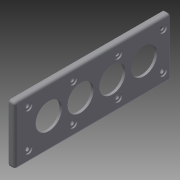
# Autodesk Inventor part: 160409 Sensor cover A_Miniature - A_Miniature - A_Miniature - A_Miniature - R23
Saved by Autodesk Inventor 2015 (Build 190159000, 159)
## iProperties
Created: 2016-02-28
Part Number: 160409 Sensor cover A_Miniature - A_Miniature - A_Miniature - A_Miniature - R23
Material: Generic
Document SubType Name: Modeling
Designer: gerbomi
Density: 1 g/cm^3
Appearance: Default
Author: gerbomi
Autodesk Inventor part; units mm, degrees
sketch "Sketch1" plane through (0, 0, 0) normal (0, 1, 0) x (-1, 0, 0)
  line L0 (2, 0) -> (102, 0)
  line L1 (104, -2) -> (104, -123)
  line L2 (102, -125) -> (2, -125)
  line L3 (0, -123) -> (0, -2)
  arc A0 (104, -2) -> (102, 0) centre (102, -2) ccw
  arc A1 (102, -125) -> (104, -123) centre (102, -123) ccw
  arc A2 (0, -123) -> (2, -125) centre (2, -123) ccw
  arc A3 (2, 0) -> (0, -2) centre (2, -2) ccw
  point P0 (0, 0)
  point P1 (104, -125)
  point P2 (0, -125)
  dimension "d0" = 104
  dimension "d1" = 125
  dimension "d2" = 2
  dimension "d3" = 2
  constraints: 8 end point, 8 point on circle, 8 tangent, 6 point on line, 4 centre point, 2 equal radius, 2 parallel, 1 horizontal, 1 perpendicular
  measures "d0" distance of point (104, -125) point (0, -125)
  measures "d1" distance of point (0, -125) point (0, 0)
  measures "d2" radius of A0
  measures "d3" radius of A3
extrude "Boîte extérieure" [suppressed]
fillet "Fillet1-Boîte extérieure" [suppressed]
ref_plane "Work Plane2 - PCB Vertical" through (0, 0, -62.5) normal (0, 0, 1) x (1, 0, 0)
ref_plane "Work Plane4 - Surface extérieure capteurs" through (0, 20.1, 0) normal (0, 1, 0) x (-1, 0, 0)
ref_plane "Work Plane6 - Fond creusé" through (0, 17, 0) normal (0, 1, 0) x (-1, 0, 0)
sketch "Sketch26" plane through (0, 20.1, 0) normal (0, 1, 0) x (-1, 0, 0)
  line L0 (16, -121) -> (36, -121)
  line L1 (47, -110) -> (47, -13)
  line L2 (36, -2) -> (16, -2)
  line L3 (5, -13) -> (5, -110)
  arc A0 (5, -110) -> (16, -121) centre (16, -110) ccw
  arc A1 (36, -121) -> (47, -110) centre (36, -110) ccw
  arc A2 (47, -13) -> (36, -2) centre (36, -13) ccw
  arc A3 (16, -2) -> (5, -13) centre (16, -13) ccw
  line L4 (0, -2) -> (0, -123) projected
  line L5 (0, -2) -> (0, -123) projected
  line L6 (104, -123) -> (104, -2) projected
  line L7 (2, -125) -> (102, -125) projected
  point P0 (0, 0)
  point P1 (47, -2)
  point P2 (47, -121)
  point P3 (5, -2)
  dimension "d158" = 42
  dimension "d159" = 119
  dimension "d160" = 11
  dimension "d161" = 5
  dimension "d186" = 4
  constraints: 8 end point, 8 point on circle, 8 tangent, 6 point on line, 4 centre point, 3 equal radius, 2 parallel, 1 horizontal, 1 perpendicular
  measures "d158" distance of point (5, -2) point (47, -2)
  measures "d159" distance of point (47, -2) point (47, -121)
  measures "d160" radius of A0
  measures "d161" distance between parallel lines of L4 L3
  measures "d186" distance between parallel lines of L7 L0
extrude "Centreur Echantillonnage actif" [suppressed]
sketch "Sketch 22" plane through (0, 17, 0) normal (0, 1, 0) x (-1, 0, 0)
  circle A0 centre (25.1, -19.83) radius 16.5
  line L0 (99, -5) -> (99, -120) projected
  line L1 (9, -5) -> (99, -5) projected
  circle A1 centre (25.1, -47.135) radius 10.5
  circle A2 centre (25.1, -72.535) radius 10.5
  circle A3 centre (25.1, -99.84) radius 16.5
  line L2 (102, 0) -> (2, 0) projected
  line L3 (0, -2) -> (0, -123) projected
  line L4 (2, -125) -> (102, -125) projected
  point P0 (0, 0)
  point P1 (99, -12.0721)
  point P2 (99, -58.79)
  point P3 (16.07, -5)
  point P4 (91.93, -5)
  dimension "d124" = 33
  dimension "d126" = 14.83
  dimension "d140" = 21
  dimension "d141" = 27.305
  dimension "d142" = 21
  dimension "d143" = 25.4
  dimension "d144" = 33
  dimension "d145" = 27.305
  dimension "d196" = 73.9
  dimension "d258" = 19.83
  dimension "d259" = 25.1
  dimension "d260" = 25.16
  constraints: 4 centre point
  measures "d124" diameter of A0
  measures "d126" distance from line of L1 A0.centre
  measures "d140" diameter of A1
  measures "d141" distance of A0.centre A1.centre
  measures "d142" diameter of A2
  measures "d143" distance of A1.centre A2.centre
  measures "d144" diameter of A3
  measures "d145" distance of A2.centre A3.centre
  measures "d196" distance from line of L0 A0.centre
  measures "d258" distance from line of L2 A0.centre
  measures "d259" distance from line of A0.centre L3
  measures "d260" distance from line of L4 A3.centre
extrude "Sensor A/Miniature or Sensoric" [suppressed]
sketch "Sketch35" plane through (0, 20.1, 0) normal (0, 1, 0) x (-1, 0, 0)
  circle A0 centre (40.5, -114) radius 1
  line L0 (47, -110) -> (47, -13) projected
  line L1 (16, -121) -> (36, -121) projected
  point P0 (0, 0)
  dimension "d235" = 2
  dimension "d244" = 6.5
  dimension "d245" = 7
  constraints: 1 centre point
  measures "d235" diameter of A0
  measures "d244" distance from line of L0 A0.centre
  measures "d245" distance from line of L1 A0.centre
extrude "Vis Centreur Chapeau" [suppressed]
pattern_linear "Rectangular Pattern3" [suppressed]
ref_plane "Work Plane10 - Chapeau ext." through (0, 25.1, 0) normal (0, 1, 0) x (-1, 0, 0)
sketch "Sketch36" plane through (0, 25.1, 0) normal (0, 1, 0) x (-1, 0, 0)
  line L0 (102, -125) -> (2, -125)
  line L1 (102, 0) -> (2, 0) projected
  line L2 (2.8, -125) -> (49.2, -125)
  line L3 (49.2, -125) -> (49.2, 0)
  line L4 (49.2, 0) -> (2.8, 0)
  line L5 (2.8, 0) -> (2.8, -125)
  line L6 (47, -110) -> (47, -13) projected
  point P0 (0, 0)
  dimension "d247" = 46.4
  dimension "d252" = 125
  constraints: 10 end point, 2 parallel, 2 point on line, 1 horizontal, 1 perpendicular
  measures "d247" distance of L4.end L3.end
  measures "d252" distance between parallel lines of L0 L1
extrude "Chapeau" add sketch "Sketch36" against normal blind 4.9
fillet "Fillet10" radius 2 8 edges at (-49.2, 25.1, -62.5) (-26, 25.1, -125) (-49.2, 22.65, -125) (-2.8, 22.65, -125) (-2.8, 25.1, -62.5) (-2.8, 22.65, 0) (-26, 25.1, 0) (-49.2, 22.65, 0)
ref_plane "Work Plane11 - Haut capteurs shields" through (0, 23.1, 0) normal (0, 1, 0) x (-1, 0, 0)
sketch "Sketch37" plane through (0, 23.1, 0) normal (0, 1, 0) x (-1, 0, 0)
  line L0 (14.5, -1.5) -> (37.5, -1.5)
  line L1 (47.5, -11.5) -> (47.5, -111.5)
  line L2 (37.5, -121.5) -> (14.5, -121.5)
  line L3 (4.5, -111.5) -> (4.5, -11.5)
  line L4 (4.8, 0) -> (47.2, 0) projected
  line L5 (2.8, -123) -> (2.8, -2) projected
  line L6 (47.2, -125) -> (4.8, -125) projected
  arc A0 (4.5, -111.5) -> (14.5, -121.5) centre (14.5, -111.5) ccw
  arc A1 (37.5, -121.5) -> (47.5, -111.5) centre (37.5, -111.5) ccw
  arc A2 (47.5, -11.5) -> (37.5, -1.5) centre (37.5, -11.5) ccw
  arc A3 (14.5, -1.5) -> (4.5, -11.5) centre (14.5, -11.5) ccw
  point P0 (0, 0)
  point P1 (4.5, -1.5)
  point P2 (47.5, -121.5)
  point P3 (47.5, -1.5)
  point P4 (4.5, -121.5)
  dimension "d254" = 43
  dimension "d255" = 120
  dimension "d257" = 1.7
  dimension "d263" = 3.5
  dimension "d264" = 10
  constraints: 8 end point, 8 point on circle, 8 point on line, 8 tangent, 4 centre point, 3 equal radius, 2 parallel, 1 horizontal, 1 perpendicular
  measures "d254" distance of point (47.5, -121.5) point (4.5, -121.5)
  measures "d255" distance of point (47.5, -1.5) point (47.5, -121.5)
  measures "d257" distance between parallel lines of L3 L5
  measures "d263" distance between parallel lines of L2 L6
  measures "d264" radius of A0
extrude "Creusement interne pour passage Centreur" cut sketch "Sketch37" against normal blind 2.9
sketch "Sketch41" plane through (0, 25.1, 0) normal (0, 1, 0) x (-1, 0, 0)
  circle A0 centre (40.5, -114) radius 1.5
  point P0 (0, 0)
  dimension "d276" = 3
  constraints: 1 centre point
  measures "d276" diameter of A0
extrude "Alesage de vissage chapeau" cut sketch "Sketch41" against normal blind 2
sketch "Sketch38" plane through (0, 23.1, 0) normal (0, 1, 0) x (-1, 0, 0)
  line L0 (47.2, -125) -> (4.8, -125) projected
  line L1 (4.8, 0) -> (47.2, 0) projected
  circle A0 centre (25.1, -97.935) radius 8.25
  circle A1 centre (25.1, -72.535) radius 8.25
  circle A2 centre (25.1, -47.135) radius 8.25
  point P0 (0, 0)
  point P1 (25.1, -99.84)
  point P2 (25.1, -19.83)
  point P3 (25.1, -21.735)
  dimension "d265" = 25.16
  dimension "d266" = 27.305
  dimension "d267" = 25.4
  dimension "d268" = 27.305
  dimension "d269" = 19.83
  dimension "d270" = 27.065
  dimension "d271" = 25.4
  dimension "d272" = 25.4
  dimension "d273" = 21.735
  dimension "d300" = 16.5
  dimension "d301" = 16.5
  dimension "d302" = 16.5
  constraints: 3 centre point, 3 coincident
  measures "d265" distance from line of point (25.1, -99.84) L0
  measures "d266" distance of point (25.1, -72.535) point (25.1, -99.84)
  measures "d267" distance of point (25.1, -47.135) point (25.1, -72.535)
  measures "d268" distance of point (25.1, -19.83) point (25.1, -47.135)
  measures "d269" distance from line of L1 point (25.1, -19.83)
  measures "d270" distance from line of point (25.1, -97.935) L0
  measures "d271" distance of point (25.1, -72.535) point (25.1, -97.935)
  measures "d272" distance of point (25.1, -21.735) point (25.1, -47.135)
  measures "d273" distance from line of L1 point (25.1, -21.735)
  measures "d300" diameter of A0
  measures "d301" diameter of A1
  measures "d302" diameter of A2
pattern_linear "Alesages de vissages chapeau" count 2 spacing 29.9 along (1, 0, 0) count 4 spacing 35.9 along (0, 0, 1) of "Alesage de vissage chapeau"
sketch "Sketch44" plane through (0, 25.1, 0) normal (0, 1, 0) x (-1, 0, 0)
  circle A0 centre (40.5, -114) radius 3
  point P0 (0, 0)
  dimension "d291" = 6
  constraints: 1 centre point
  measures "d291" diameter of A0
extrude "Epaulement tête de vis" cut sketch "Sketch44" against normal blind 1
pattern_linear "Epaulements tête de vis" count 2 spacing 29.9 along (1, 0, 0) count 4 spacing -35.9 along (0, 0, -1) of "Epaulement tête de vis"
sketch "Sketch45" plane through (0, 23.1, 0) normal (0, 1, 0) x (-1, 0, 0)
  circle A0 centre (25.1, -97.935) radius 10.5
  circle A1 centre (25.1, -72.535) radius 10.5
  circle A2 centre (25.1, -47.135) radius 10.5
  circle A3 centre (25.1, -21.735) radius 10.5
  point P0 (0, 0)
  dimension "d303" = 21
  dimension "d304" = 21
  dimension "d305" = 21
  dimension "d308" = 21
  constraints: 4 centre point
  measures "d303" diameter of A0
  measures "d304" diameter of A1
  measures "d305" diameter of A2
  measures "d308" diameter of A3
extrude "ALesages capteurs" cut sketch "Sketch45" along normal blind 2
body "Solid1"
